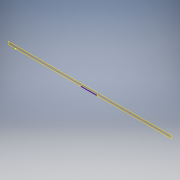
# Autodesk Inventor part: Back Plate
Saved by Autodesk Inventor 2016 (Build 200138000, 138)
## iProperties
Created: 2016-04-23
Part Number: Back Plate
Material: Generic
Document SubType Name: Modeling
Designer: Scott
Density: 1 g/cm^3
Appearance: Default
Author: Scott
Autodesk Inventor part; units mm, degrees
ref_plane "YZ Plane" through (0, 0, 0) normal (1, 0, 0) x (0, 1, 0)
ref_plane "XZ Plane" through (0, 0, 0) normal (0, 1, 0) x (-1, 0, 0)
ref_plane "XY Plane" through (0, 0, 0) normal (0, 0, 1) x (1, 0, 0)
ref_plane "Work Plane1" through (0, 0, 0) normal (0, 0, 1) x (1, 0, 0)
sketch "Sketch1" plane through (0, 0, 0) normal (0, 0, 1) x (1, 0, 0)
  line L0 (154.6225, 0) -> (150.1775, 0) projected
  line L1 (192.7225, 0) -> (188.2775, 0) projected
  line L2 (152.4, 0) -> (190.5, 0)
  line L3 (171.45, 0) -> (171.45, -267.8176)
  line L4 (139.7, -3.7338) -> (203.2, -3.7338)
  line L5 (203.2, -3.7338) -> (203.2, -264.0838)
  line L6 (203.2, -264.0838) -> (139.7, -264.0838)
  line L7 (139.7, -264.0838) -> (139.7, -3.7338)
  line L8 (139.7, -3.7338) -> (203.2, -264.0838) construction
  line L9 (203.2, -3.7338) -> (139.7, -264.0838) construction
  line L10 (139.7, -264.0838) -> (139.7, -251.3838)
  circle A0 centre (152.4, -251.3838) radius 2.2225
  line L11 (203.2, -264.0838) -> (203.2, -251.3838)
  circle A1 centre (190.5, -251.3838) radius 2.2225
  circle A2 centre (152.4, -225.9838) radius 2.2225
  circle A3 centre (190.5, -225.9838) radius 2.2225
  line L12 (139.7, -133.9088) -> (152.4, -133.9088)
  line L13 (171.45, -267.8176) -> (171.45, 0)
  line L14 (139.7, -264.0838) -> (203.2, -3.7338) construction
  line L15 (203.2, -264.0838) -> (139.7, -3.7338) construction
  circle A4 centre (152.4, -16.4338) radius 2.2225
  circle A5 centre (190.5, -16.4338) radius 2.2225
  circle A6 centre (152.4, -41.8338) radius 2.2225
  circle A7 centre (190.5, -41.8338) radius 2.2225
  point P0 (0, 0)
  point P1 (171.45, -133.9088)
  dimension "d0" = 267.8176
  dimension "d1" = 63.5
  dimension "d2" = 260.35
  dimension "d3" = 12.7
  dimension "d5" = 4.445
  dimension "d7" = 4.445
  dimension "d10" = 25.4
  constraints: 28 end point, 10 symmetric about line, 8 centre point, 7 midpoint, 2 horizontal, 2 parallel, 2 point on line, 2 vertical, 1 perpendicular, 8 other
  measures "d0" distance of L3.start L3.end
  measures "d1" distance of L5.end L6.end
  measures "d2" distance of L4.end L5.end
  measures "d3" distance of L6.end L10.end
  measures "d5" diameter of A0
  measures "d7" diameter of A1
  measures "d10" distance of A0.centre A2.centre
extrude "Extrusion1" add sketch "Sketch1" against normal blind 6.096
body "Solid1"
